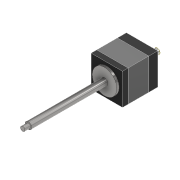
# Autodesk Inventor part: duzy_silnik
Saved by Autodesk Inventor 2021 (Build 250183000, 183)
## iProperties
Created: 2022-05-17
Part Number: duzy_silnik
Material: Generic
Document SubType Name: Modeling
Designer: agnpi
Density: 1 g/cm^3
Appearance: Default
Author: agnpi
Autodesk Inventor part; units mm, degrees
ref_plane "YZ Plane" through (0, 0, 0) normal (1, 0, 0) x (0, 1, 0)
ref_plane "XZ Plane" through (0, 0, 0) normal (0, 1, 0) x (-1, 0, 0)
ref_plane "XY Plane" through (0, 0, 0) normal (0, 0, 1) x (1, 0, 0)
sketch "Sketch1" plane through (0, 0, 0) normal (0, 0, 1) x (1, 0, 0)
  line L0 (0, -19.6) -> (0, 19.6) projected
  line L1 (-19.6, 0) -> (19.6, 0) projected
  line L2 (-14, 14) -> (14, 14)
  line L3 (14, 14) -> (14, -14)
  line L4 (14, -14) -> (-14, -14)
  line L5 (-14, -14) -> (-14, 14)
  line L6 (-14, 14) -> (14, -14) construction
  line L7 (14, 14) -> (-14, -14) construction
  point P0 (0, 0)
  dimension "d0" = 28
  dimension "d1" = 28
  constraints: 12 end point, 2 midpoint, 2 parallel, 1 horizontal, 1 perpendicular
  measures "d0" distance of L3.end L4.end
  measures "d1" distance of L2.end L3.end
extrude "Extrusion1" add sketch "Sketch1" along normal blind 8
sketch "Sketch2" plane through (0, 0, 8) normal (0, 0, 1) x (1, 0, 0)
  line L0 (-14, -14) -> (14, -14) projected
  line L1 (-14, 14) -> (14, 14)
  line L2 (14, 14) -> (14, -14)
  line L3 (14, -14) -> (-14, -14)
  line L4 (-14, -14) -> (-14, 14)
  line L5 (-14, 14) -> (14, -14) construction
  line L6 (14, 14) -> (-14, -14) construction
  point P0 (0, 0)
  constraints: 12 end point, 2 midpoint, 2 parallel, 1 horizontal, 1 perpendicular
extrude "Extrusion2" add sketch "Sketch2" along normal blind 18.5 separate body
sketch "Sketch3" plane through (0, 0, 26.5) normal (0, 0, 1) x (1, 0, 0)
  line L0 (-14, -14) -> (14, -14) projected
  line L1 (-14, 14) -> (14, 14)
  line L2 (14, 14) -> (14, -14)
  line L3 (14, -14) -> (-14, -14)
  line L4 (-14, -14) -> (-14, 14)
  line L5 (-14, 14) -> (14, -14) construction
  line L6 (14, 14) -> (-14, -14) construction
  point P0 (0, 0)
  constraints: 12 end point, 2 midpoint, 2 parallel, 1 horizontal, 1 perpendicular
extrude "Extrusion3" add sketch "Sketch3" along normal blind 5 separate body
sketch "Sketch4" plane through (0, 0, 31.5) normal (0, 0, 1) x (1, 0, 0)
  circle A0 centre (0, 0) radius 11
  dimension "d8" = 22
  constraints: 1 centre point, 1 coincident
  measures "d8" diameter of A0
extrude "Extrusion4" add sketch "Sketch4" along normal blind 2 separate body
sketch "Sketch6" plane through (0, 0, 0) normal (0, 0, -1) x (-1, 0, 0)
  circle A0 centre (0, 0) radius 2.5
  dimension "d14" = 5
  constraints: 1 centre point, 1 coincident
  measures "d14" diameter of A0
extrude "Extrusion6" add sketch "Sketch6" along normal blind 13.5 separate body
sketch "Sketch7" plane through (0, 0, 33.5) normal (0, 0, 1) x (1, 0, 0)
  circle A0 centre (0, 0) radius 3
  dimension "d17" = 6
  constraints: 1 centre point, 1 coincident
  measures "d17" diameter of A0
extrude "Extrusion7" add sketch "Sketch7" along normal blind 68 bodies 4
sketch "Sketch8" plane through (0, 0, 101.5) normal (0, 0, 1) x (1, 0, 0)
  circle A0 centre (0, 0) radius 2
  dimension "d20" = 4
  constraints: 1 centre point, 1 coincident
  measures "d20" diameter of A0
extrude "Extrusion8" add sketch "Sketch8" along normal blind 5 bodies 4
body "Solid1"
body "Solid2"
body "Solid3"
body "Solid4"
body "Solid6"
